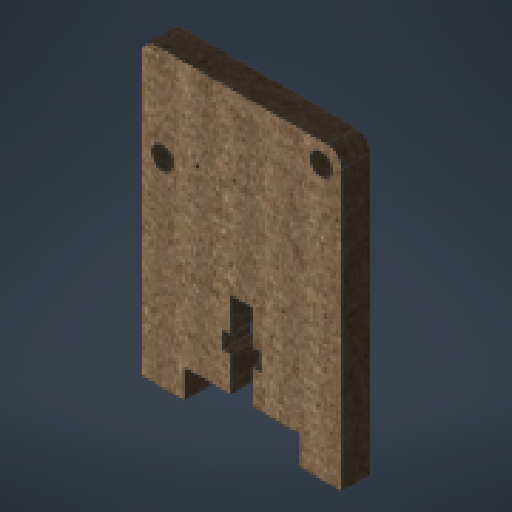
# Autodesk Inventor part: SwitchHolder_Bottom_V3
Saved by Autodesk Inventor 2024.1 (Build 281209000, 209)
## iProperties
Created: 2022-12-01
Part Number: SwitchHolder_Bottom_V3
Material: MDF Medium Density Fiberboard
Document SubType Name: Modeling
Designer: jaege
Density: 0.8 g/cm^3
Appearance: Cardboard - Corrugated
Author: jaege
Autodesk Inventor part; units mm, degrees
ref_plane "YZ Plane" through (0, 0, 0) normal (1, 0, 0) x (0, 1, 0)
ref_plane "XZ Plane" through (0, 0, 0) normal (0, 1, 0) x (-1, 0, 0)
ref_plane "XY Plane" through (0, 0, 0) normal (0, 0, 1) x (1, 0, 0)
sketch "Sketch1" plane through (0, 0, 0) normal (0, 0, 1) x (1, 0, 0)
  line L0 (-14, 0) -> (14, 0)
  line L1 (14, 0) -> (14, 16)
  line L2 (14, 16) -> (-14, 16)
  line L3 (-14, 16) -> (-14, 0)
  circle A0 centre (-11.1, 2.85) radius 1.55
  circle A1 centre (11.1, 13.15) radius 1.55
  line L4 (-11.1, 2.85) -> (-14, 2.85) construction
  line L5 (11.1, 13.15) -> (14, 13.15) construction
  line L6 (11.1, 13.15) -> (11.1, 16) construction
  line L7 (-11.1, 2.85) -> (-11.1, 0) construction
  line L8 (-14, 0) -> (14, 0) construction
  line L9 (14, 0) -> (14, -24.4)
  line L10 (14, -24.4) -> (8, -24.4) construction
  line L11 (-14, -24.4) -> (-14, 0)
  line L12 (-14, -24.4) -> (-8, -24.4) construction
  line L13 (-8, -24.4) -> (-8, -28.4)
  line L14 (-8, -28.4) -> (-14, -28.4)
  line L15 (-14, -28.4) -> (-14, -24.4)
  line L16 (14, -24.4) -> (8, -24.4) construction
  line L17 (8, -24.4) -> (8, -28.4)
  line L18 (8, -28.4) -> (14, -28.4)
  line L19 (14, -28.4) -> (14, -24.4)
  line L20 (-8, -24.4) -> (-14, -24.4) construction
  line L21 (8, -24.4) -> (-8, -24.4)
  point P0 (0, 0)
  point P1 (0, 0)
  point P2 (14, 0)
  point P3 (14, 0)
  dimension "d0" = 3.1
  dimension "d1" = 22.2
  dimension "d2" = 10.3
  dimension "d3" = 16
  dimension "d4" = 28
  dimension "d5" = 40.4
  dimension "d8" = 6
  dimension "d9" = 6
  dimension "d10" = 4
  constraints: 44 end point, 12 parallel, 8 perpendicular, 5 point on line, 4 horizontal, 2 centre point, 1 coincident, 1 collinear, 1 equal radius, 1 horizontal alignment, 1 midpoint
  measures "d0" diameter of A1
  measures "d1" horizontal distance of L5.start L4.start
  measures "d2" vertical distance of L5.start L4.start
  measures "d3" distance of L0.end L1.end
  measures "d4" distance of L1.end L2.end
  measures "d5" distance between parallel lines of L2 L10
  measures "d8" distance of L13.end L14.end
  measures "d9" distance of L18.end L17.end
  measures "d10" distance of L18.end L9.end
extrude "Extrusion1" add sketch "Sketch1" along normal blind 4
sketch "Sketch2" plane through (0, 0, 4) normal (0, 0, 1) x (1, 0, 0)
  line L0 (14, -28.4) -> (14, 16) construction
  line L1 (14, 16) -> (-14, 16) construction
  line L2 (-14, 16) -> (-14, -28.4) construction
  line L3 (-14, -28.4) -> (-8, -28.4) construction
  line L4 (-8, -28.4) -> (-8, -24.4) construction
  line L5 (-8, -24.4) -> (8, -24.4) construction
  line L6 (8, -24.4) -> (8, -28.4) construction
  line L7 (8, -28.4) -> (14, -28.4) construction
  circle A0 centre (-11.1, 2.85) radius 1.55 construction
  circle A1 centre (11.1, 13.15) radius 1.55 construction
  line L8 (-1.5, -24.4) -> (1.5, -24.4)
  line L9 (1.5, -24.4) -> (1.5, -12.4)
  line L10 (1.5, -12.4) -> (-1.5, -12.4)
  line L11 (-1.5, -12.4) -> (-1.5, -24.4)
  line L12 (-2.7, -19.6) -> (2.7, -19.6)
  line L13 (2.7, -19.6) -> (2.7, -17.2)
  line L14 (2.7, -17.2) -> (-2.7, -17.2)
  line L15 (-2.7, -17.2) -> (-2.7, -19.6)
  point P0 (0, 0)
  point P1 (-2.7, -18.4)
  point P2 (-1.5, -18.4)
  point P3 (0, -17.2)
  point P4 (0, -12.4)
  point P5 (0, -24.4)
  point P6 (0, -24.4)
  point P7 (-1.5, -19.6)
  point P8 (1.5, -19.6)
  point P9 (1.5, -17.2)
  point P10 (-1.5, -17.2)
  dimension "d11" = 3
  dimension "d12" = 2.4
  dimension "d13" = 5.4
  dimension "d14" = 12
  constraints: 16 end point, 6 midpoint, 4 parallel, 2 horizontal, 2 perpendicular, 1 coincident, 1 horizontal alignment, 1 point on line, 1 vertical alignment
  measures "d11" distance of L9.end L10.end
  measures "d12" distance of L14.end L12.start
  measures "d13" distance of L13.end L14.end
  measures "d14" distance of L8.end L9.end
extrude "Extrusion2" cut sketch "Sketch2" against normal up to next
fillet "Fillet1" radius 2 2 edges at (14, 16, 2) (-14, 16, 2)
body "Solid1"
